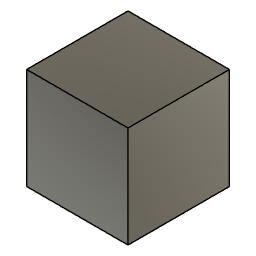
wheel (Autodesk Fusion 360 archive; units mm, degrees)
design "휠 기준점"
Autodesk Fusion 360 part; units mm, degrees
sketch "스케치1" plane through (0, 0, 0) normal (0, 0, 1) x (1, 0, 0)
  line L0 (0, 0) -> (-3, 0)
  line L1 (-3, 0) -> (-3, 3)
  line L2 (-3, 3) -> (0, 3)
  line L3 (0, 3) -> (0, 0)
  dimension "d1" = 3
  dimension "d2" = 3
  constraint horizontal L0
  constraint vertical L1
  constraint horizontal L2
  constraint vertical L3
  constraint coincident L0.start L3.end
  measures "d1" distance of L0.start L0.end
  measures "d2" distance of L0.start L2.end
extrude "돌출1" add sketch "스케치1" along normal blind 3

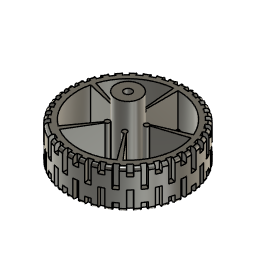
design "휠"
Autodesk Fusion 360 part; units mm, degrees
sketch "스케치1" plane through (0, 0, 0) normal (0, 0, 1) x (1, 0, 0)
  circle A0 centre (0, 0) radius 62.5
  dimension "d1" = 125
  constraint coincident A0.centre origin
  measures "d1" diameter of A0
extrude "돌출1" add sketch "스케치1" along normal blind 40
sketch "스케치2" plane through (0, 0, 40) normal (0, 0, 1) x (-1, 0, 0)
  circle A0 centre (0, 0) radius 62.5
  circle A1 centre (0, 0) radius 13
  dimension "d4" = 26
  constraint coincident A0.centre A1.centre
  measures "d4" diameter of A1
extrude "돌출2" add sketch "스케치2" along normal blind 25.5 contours A1
sketch "스케치3" plane through (0, 0, 65.5) normal (0, 0, 1) x (-1, 0, 0)
  circle A0 centre (0, 0) radius 13
  circle A1 centre (0, 0) radius 4
  dimension "d7" = 8
  constraint coincident A0.centre A1.centre
  measures "d7" diameter of A1
extrude "돌출3" cut sketch "스케치3" against normal blind 20.5 contours A1
sketch "스케치6" plane through (0, 0, 0) normal (0, 0, 1) x (1, 0, 0)
  circle A0 centre (0, 0) radius 18
  circle A1 centre (0, 0) radius 21
  circle A2 centre (0, 0) radius 55
  circle A3 centre (0, 0) radius 52.5
  line L0 (0, 0) -> (0, 52.5)
  line L1 (0, 0) -> (49.9305, 16.2234)
  line L2 (0, 0) -> (30.8587, -42.4734)
  line L3 (0, 0) -> (-30.8587, -42.4734)
  line L4 (0, 0) -> (-49.9305, 16.2234)
  line L5 (0, 21) -> (10, 21)
  line L6 (10, 21) -> (0, 52.5)
  line L7 (10, 21) -> (37.4155, 36.8284)
  line L8 (10, 21) -> (40.9959, 21) construction
  line L9 (19.9722, 6.4894) -> (23.0624, -3.0212)
  line L10 (23.0624, -3.0212) -> (49.9305, 16.2234)
  line L11 (23.0624, -3.0212) -> (46.5879, -24.2037)
  line L12 (12.3435, -16.9894) -> (4.2533, -22.8672)
  line L13 (4.2533, -22.8672) -> (30.8587, -42.4734)
  line L14 (4.2533, -22.8672) -> (-8.6226, -51.7871)
  line L15 (-12.3435, -16.9894) -> (-20.4337, -11.1115)
  line L16 (-20.4337, -11.1115) -> (-30.8587, -42.4734)
  line L17 (-20.4337, -11.1115) -> (-51.917, -7.8025)
  line L18 (-19.9722, 6.4894) -> (-16.882, 15.9999)
  line L19 (-16.882, 15.9999) -> (-49.9305, 16.2234)
  line L20 (-16.882, 15.9999) -> (-23.4638, 46.9649)
  line L21 (-16.882, 15.9999) -> (14.7747, 15.9999) construction
  dimension "d41" = 108
  dimension "d46" = 30
  constraint coincident A0.centre A1.centre
  constraint concentric A0 A2
  constraint coincident A3 L0.end
  constraint vertical L0
  constraint coincident A3 L1.end
  constraint coincident A3 L2.end
  constraint coincident A3 L3.end
  constraint coincident A3 L4.end
  constraint coincident L0 L5.start
  constraint coincident A1 L5.start
  constraint perpendicular L0 L5
  constraint horizontal L8
  constraint coincident A3 L7.end
  constraint coincident A1 L9.start
  constraint coincident L1 L9.start
  constraint tangent A1 L9
  constraint coincident A3 L11.end
  constraint coincident A1 L12.start
  constraint coincident L2 L12.start
  constraint tangent A1 L12
  constraint coincident A3 L14.end
  constraint coincident L3 L15.start
  constraint coincident A1 L15.start
  constraint perpendicular L3 L15
  constraint coincident A3 L17.end
  constraint coincident L4 L18.start
  constraint coincident A1 L18.start
  constraint perpendicular L4 L18
  constraint horizontal L21
  constraint coincident A3 L20.end
  measures "d41" angle of L0 L1
  measures "d46" angle of L7 L8
extrude "돌출6" cut sketch "스케치6" along normal blind 75 contours A3 L10 L11 | A3 L13 L14 | A3 L6 L7 | A3 L16 L17 | A3 L19 L20
extrude "돌출7" add sketch "스케치6" against normal blind 1 contours A0 L1 L2 | A0 L0 L1 | A0 L2 L3 | A0 L0 L4 | A0 L3 L4
fillet "모깎기1" radius 0.5 1 edges at (-16.7819, 6.5091, -1)
sketch "스케치7" plane through (0, 0, 0) normal (0, 0, -1) x (1, 0, 0)
  circle A0 centre (0, 0) radius 18
  line L0 (30.8587, 42.4734) -> (4.2533, 22.8672)
  line L1 (4.2533, 22.8672) -> (-8.6226, 51.7871)
  arc A1 (30.8587, 42.4734) -> (-8.6226, 51.7871) centre (0, 0) ccw
  line L2 (49.9305, -16.2234) -> (23.0624, 3.0212)
  line L3 (23.0624, 3.0212) -> (46.5879, 24.2037)
  arc A2 (49.9305, -16.2234) -> (46.5879, 24.2037) centre (0, 0) ccw
  line L4 (-49.9305, -16.2234) -> (-16.882, -15.9999)
  line L5 (-16.882, -15.9999) -> (-23.4638, -46.9649)
  arc A3 (-49.9305, -16.2234) -> (-23.4638, -46.9649) centre (0, 0) ccw
  line L6 (0, -52.5) -> (10, -21)
  line L7 (10, -21) -> (37.4155, -36.8284)
  arc A4 (0, -52.5) -> (37.4155, -36.8284) centre (0, 0) ccw
  line L8 (-30.8587, 42.4734) -> (-20.4337, 11.1115)
  line L9 (-20.4337, 11.1115) -> (-51.917, 7.8025)
  arc A5 (-30.8587, 42.4734) -> (-51.917, 7.8025) centre (0, 0) ccw
  circle A6 centre (0, 0) radius 62.5
  circle A7 centre (0, 0) radius 57.5
  circle A8 centre (0, 0) radius 62.5
  line L10 (0, 0) -> (-1.368, 1.8829)
  line L11 (0, 0) -> (-30.8587, 42.4734)
  line L12 (-30.8587, 42.4734) -> (-36.7366, 50.5636)
  line L13 (-34.4431, 39.6223) -> (-41.0037, 47.1693)
  line L14 (-37.7653, 36.4696) -> (-44.9587, 43.4161)
  line L15 (-40.8002, 33.0393) -> (-48.5716, 39.3325)
  line L16 (-43.5245, 29.3576) -> (-51.8148, 34.9496)
  line L17 (-45.9175, 25.4525) -> (-54.6637, 30.3006)
  line L18 (-47.9611, 21.3537) -> (-57.0966, 25.421)
  line L19 (-49.6397, 17.0923) -> (-59.0949, 20.348)
  line L20 (-50.9405, 12.7009) -> (-60.6435, 15.1201)
  line L21 (-51.8536, 8.2128) -> (-61.7305, 9.7772)
  line L22 (-52.3721, 3.6622) -> (-62.3478, 4.3598)
  line L23 (-52.492, -0.9163) -> (-62.4905, -1.0908)
  line L24 (-52.2124, -5.4877) -> (-62.1576, -6.533)
  line L25 (-51.5354, -10.0175) -> (-61.3517, -11.9256)
  line L26 (-50.4662, -14.471) -> (-60.0789, -17.2273)
  line L27 (-49.013, -18.8143) -> (-58.3488, -22.398)
  line L28 (-47.1867, -23.0145) -> (-56.1746, -27.3982)
  line L29 (-45.0013, -27.0395) -> (-53.573, -32.1899)
  line L30 (-42.4734, -30.8587) -> (-50.5636, -36.7366)
  line L31 (-39.6223, -34.4431) -> (-47.1693, -41.0037)
  line L32 (-36.4696, -37.7653) -> (-43.4161, -44.9587)
  line L33 (-33.0393, -40.8002) -> (-39.3325, -48.5716)
  line L34 (-29.3576, -43.5245) -> (-34.9496, -51.8148)
  line L35 (-25.4525, -45.9175) -> (-30.3006, -54.6637)
  line L36 (-21.3537, -47.9611) -> (-25.421, -57.0966)
  line L37 (-17.0923, -49.6397) -> (-20.348, -59.0949)
  line L38 (-12.7009, -50.9405) -> (-15.1201, -60.6435)
  line L39 (-8.2128, -51.8536) -> (-9.7772, -61.7305)
  line L40 (-3.6622, -52.3721) -> (-4.3598, -62.3478)
  line L41 (0.9163, -52.492) -> (1.0908, -62.4905)
  line L42 (5.4877, -52.2124) -> (6.533, -62.1576)
  line L43 (10.0175, -51.5354) -> (11.9256, -61.3517)
  line L44 (14.471, -50.4662) -> (17.2273, -60.0789)
  line L45 (18.8143, -49.013) -> (22.398, -58.3488)
  line L46 (23.0145, -47.1867) -> (27.3982, -56.1746)
  line L47 (27.0395, -45.0013) -> (32.1899, -53.573)
  line L48 (30.8587, -42.4734) -> (36.7366, -50.5636)
  line L49 (34.4431, -39.6223) -> (41.0037, -47.1693)
  line L50 (37.7653, -36.4696) -> (44.9587, -43.4161)
  line L51 (40.8002, -33.0393) -> (48.5716, -39.3325)
  line L52 (43.5245, -29.3576) -> (51.8148, -34.9496)
  line L53 (45.9175, -25.4525) -> (54.6637, -30.3006)
  line L54 (47.9611, -21.3537) -> (57.0966, -25.421)
  line L55 (49.6397, -17.0923) -> (59.0949, -20.348)
  line L56 (50.9405, -12.7009) -> (60.6435, -15.1201)
  line L57 (51.8536, -8.2128) -> (61.7305, -9.7772)
  line L58 (52.3721, -3.6622) -> (62.3478, -4.3598)
  line L59 (52.492, 0.9163) -> (62.4905, 1.0908)
  line L60 (52.2124, 5.4877) -> (62.1576, 6.533)
  line L61 (51.5354, 10.0175) -> (61.3517, 11.9256)
  line L62 (50.4662, 14.471) -> (60.0789, 17.2273)
  line L63 (49.013, 18.8143) -> (58.3488, 22.398)
  line L64 (47.1867, 23.0145) -> (56.1746, 27.3982)
  line L65 (45.0013, 27.0395) -> (53.573, 32.1899)
  line L66 (42.4734, 30.8587) -> (50.5636, 36.7366)
  line L67 (39.6223, 34.4431) -> (47.1693, 41.0037)
  line L68 (36.4696, 37.7653) -> (43.4161, 44.9587)
  line L69 (33.0393, 40.8002) -> (39.3325, 48.5716)
  line L70 (29.3576, 43.5245) -> (34.9496, 51.8148)
  line L71 (25.4525, 45.9175) -> (30.3006, 54.6637)
  line L72 (21.3537, 47.9611) -> (25.421, 57.0966)
  line L73 (17.0923, 49.6397) -> (20.348, 59.0949)
  line L74 (12.7009, 50.9405) -> (15.1201, 60.6435)
  line L75 (8.2128, 51.8536) -> (9.7772, 61.7305)
  line L76 (3.6622, 52.3721) -> (4.3598, 62.3478)
  line L77 (-0.9163, 52.492) -> (-1.0908, 62.4905)
  line L78 (-5.4877, 52.2124) -> (-6.533, 62.1576)
  line L79 (-10.0175, 51.5354) -> (-11.9256, 61.3517)
  line L80 (-14.471, 50.4662) -> (-17.2273, 60.0789)
  line L81 (-18.8143, 49.013) -> (-22.398, 58.3488)
  line L82 (-23.0145, 47.1867) -> (-27.3982, 56.1746)
  line L83 (-27.0395, 45.0013) -> (-32.1899, 53.573)
  dimension "d61" = 115
  dimension "d62" = 125
  dimension "d64" = 360
  constraint coincident A0.centre A1.centre
  constraint concentric A7 A8
  constraint coincident L8.start A5.start
  constraint coincident A8 L12.end
  constraint parallel L11 L12
  measures "d61" diameter of A7
  measures "d62" diameter of A8
fillet "모깎기2" radius 3 1 edges at (-58.2705, -22.601, 0)
extrude "돌출8" cut sketch "스케치7" against normal blind 20 contours A6 A7 A8 L71 L72 | A6 A7 A8 L67 L68 | A6 A7 A8 L79 L80 | A6 A7 A8 L75 L76 | A6 A7 A8 L63 L64 | A6 A7 A8 L12 L83 | A6 A7 A8 L59 L60 | A6 A7 A8 L15 L16 | A6 A7 A8 L55 L56 | A6 A7 A8 L19 L20 | A6 A7 A8 L23 L24 | A6 A7 A8 L51 L52 | A6 A7 A8 L27 L28 | A6 A7 A8 L47 L48 | A6 A7 A8 L31 L32 | A6 A7 A8 L43 L44 | A6 A7 A8 L35 L36 | A6 A7 A8 L39 L40
extrude "돌출9" cut sketch "스케치7" against normal blind 8 contours A6 A7 A8 L69 L70 | A6 A7 A8 L77 L78 | A6 A7 A8 L73 L74 | A6 A7 A8 L65 L66 | A6 A7 A8 L81 L82 | A6 A7 A8 L61 L62 | A6 A7 A8 L13 L14 | A6 A7 A8 L17 L18 | A6 A7 A8 L21 L22 | A6 A7 A8 L57 L58 | A6 A7 A8 L53 L54 | A6 A7 A8 L25 L26 | A6 A7 A8 L49 L50 | A6 A7 A8 L29 L30 | A6 A7 A8 L45 L46 | A6 A7 A8 L33 L34 | A6 A7 A8 L41 L42 | A6 A7 A8 L37 L38
sketch "스케치8" plane through (0, 0, 40) normal (0, 0, 1) x (-1, 0, 0)
  line L0 (-4.2533, 22.8672) -> (-30.8587, 42.4734)
  arc A0 (8.6226, 51.7871) -> (-30.8587, 42.4734) centre (0, 0) ccw
  line L1 (8.6226, 51.7871) -> (-4.2533, 22.8672)
  line L2 (-23.0624, 3.0212) -> (-49.9305, -16.2234)
  arc A1 (-46.5879, 24.2037) -> (-49.9305, -16.2234) centre (0, 0) ccw
  line L3 (-46.5879, 24.2037) -> (-23.0624, 3.0212)
  line L4 (16.882, -15.9999) -> (49.9305, -16.2234)
  arc A2 (23.4638, -46.9649) -> (49.9305, -16.2234) centre (0, 0) ccw
  line L5 (23.4638, -46.9649) -> (16.882, -15.9999)
  line L6 (-10, -21) -> (0, -52.5)
  arc A3 (-37.4155, -36.8284) -> (0, -52.5) centre (0, 0) ccw
  line L7 (-37.4155, -36.8284) -> (-10, -21)
  line L8 (20.4337, 11.1115) -> (30.8587, 42.4734)
  arc A4 (51.917, 7.8025) -> (30.8587, 42.4734) centre (0, 0) ccw
  line L9 (51.917, 7.8025) -> (20.4337, 11.1115)
  circle A5 centre (0, 0) radius 13
  circle A6 centre (0, 0) radius 62.5
  circle A7 centre (0, 0) radius 62.5
  circle A8 centre (0, 0) radius 57.5
  line L10 (0, 0) -> (0, -1.8263)
  line L11 (0, -1.8263) -> (23.4638, -46.9649)
  line L12 (0, 0) -> (30.8587, 42.4734)
  line L13 (30.8587, 42.4734) -> (36.7366, 50.5636)
  line L14 (27.0395, 45.0013) -> (32.1899, 53.573)
  line L15 (23.0145, 47.1867) -> (27.3982, 56.1746)
  line L16 (18.8143, 49.013) -> (22.398, 58.3488)
  line L17 (14.471, 50.4662) -> (17.2273, 60.0789)
  line L18 (10.0175, 51.5354) -> (11.9256, 61.3517)
  line L19 (5.4877, 52.2124) -> (6.533, 62.1576)
  line L20 (0.9163, 52.492) -> (1.0908, 62.4905)
  line L21 (-3.6622, 52.3721) -> (-4.3598, 62.3478)
  line L22 (-8.2128, 51.8536) -> (-9.7772, 61.7305)
  line L23 (-12.7009, 50.9405) -> (-15.1201, 60.6435)
  line L24 (-17.0923, 49.6397) -> (-20.348, 59.0949)
  line L25 (-21.3537, 47.9611) -> (-25.421, 57.0966)
  line L26 (-25.4525, 45.9175) -> (-30.3006, 54.6637)
  line L27 (-29.3576, 43.5245) -> (-34.9496, 51.8148)
  line L28 (-33.0393, 40.8002) -> (-39.3325, 48.5716)
  line L29 (-36.4696, 37.7653) -> (-43.4161, 44.9587)
  line L30 (-39.6223, 34.4431) -> (-47.1693, 41.0037)
  line L31 (-42.4734, 30.8587) -> (-50.5636, 36.7366)
  line L32 (-45.0013, 27.0395) -> (-53.573, 32.1899)
  line L33 (-47.1867, 23.0145) -> (-56.1746, 27.3982)
  line L34 (-49.013, 18.8143) -> (-58.3488, 22.398)
  line L35 (-50.4662, 14.471) -> (-60.0789, 17.2273)
  line L36 (-51.5354, 10.0175) -> (-61.3517, 11.9256)
  line L37 (-52.2124, 5.4877) -> (-62.1576, 6.533)
  line L38 (-52.492, 0.9163) -> (-62.4905, 1.0908)
  line L39 (-52.3721, -3.6622) -> (-62.3478, -4.3598)
  line L40 (-51.8536, -8.2128) -> (-61.7305, -9.7772)
  line L41 (-50.9405, -12.7009) -> (-60.6435, -15.1201)
  line L42 (-49.6397, -17.0923) -> (-59.0949, -20.348)
  line L43 (-47.9611, -21.3537) -> (-57.0966, -25.421)
  line L44 (-45.9175, -25.4525) -> (-54.6637, -30.3006)
  line L45 (-43.5245, -29.3576) -> (-51.8148, -34.9496)
  line L46 (-40.8002, -33.0393) -> (-48.5716, -39.3325)
  line L47 (-37.7653, -36.4696) -> (-44.9587, -43.4161)
  line L48 (-34.4431, -39.6223) -> (-41.0037, -47.1693)
  line L49 (-30.8587, -42.4734) -> (-36.7366, -50.5636)
  line L50 (-27.0395, -45.0013) -> (-32.1899, -53.573)
  line L51 (-23.0145, -47.1867) -> (-27.3982, -56.1746)
  line L52 (-18.8143, -49.013) -> (-22.398, -58.3488)
  line L53 (-14.471, -50.4662) -> (-17.2273, -60.0789)
  line L54 (-10.0175, -51.5354) -> (-11.9256, -61.3517)
  line L55 (-5.4877, -52.2124) -> (-6.533, -62.1576)
  line L56 (-0.9163, -52.492) -> (-1.0908, -62.4905)
  line L57 (3.6622, -52.3721) -> (4.3598, -62.3478)
  line L58 (8.2128, -51.8536) -> (9.7772, -61.7305)
  line L59 (12.7009, -50.9405) -> (15.1201, -60.6435)
  line L60 (17.0923, -49.6397) -> (20.348, -59.0949)
  line L61 (21.3537, -47.9611) -> (25.421, -57.0966)
  line L62 (25.4525, -45.9175) -> (30.3006, -54.6637)
  line L63 (29.3576, -43.5245) -> (34.9496, -51.8148)
  line L64 (33.0393, -40.8002) -> (39.3325, -48.5716)
  line L65 (36.4696, -37.7653) -> (43.4161, -44.9587)
  line L66 (39.6223, -34.4431) -> (47.1693, -41.0037)
  line L67 (42.4734, -30.8587) -> (50.5636, -36.7366)
  line L68 (45.0013, -27.0395) -> (53.573, -32.1899)
  line L69 (47.1867, -23.0145) -> (56.1746, -27.3982)
  line L70 (49.013, -18.8143) -> (58.3488, -22.398)
  line L71 (50.4662, -14.471) -> (60.0789, -17.2273)
  line L72 (51.5354, -10.0175) -> (61.3517, -11.9256)
  line L73 (52.2124, -5.4877) -> (62.1576, -6.533)
  line L74 (52.492, -0.9163) -> (62.4905, -1.0908)
  line L75 (52.3721, 3.6622) -> (62.3478, 4.3598)
  line L76 (51.8536, 8.2128) -> (61.7305, 9.7772)
  line L77 (50.9405, 12.7009) -> (60.6435, 15.1201)
  line L78 (49.6397, 17.0923) -> (59.0949, 20.348)
  line L79 (47.9611, 21.3537) -> (57.0966, 25.421)
  line L80 (45.9175, 25.4525) -> (54.6637, 30.3006)
  line L81 (43.5245, 29.3576) -> (51.8148, 34.9496)
  line L82 (40.8002, 33.0393) -> (48.5716, 39.3325)
  line L83 (37.7653, 36.4696) -> (44.9587, 43.4161)
  line L84 (34.4431, 39.6223) -> (41.0037, 47.1693)
  dimension "d74" = 360
  constraint coincident A0.centre A1.centre
  constraint concentric A7 A8
  constraint vertical L10
  constraint coincident A2.start L5.start
  constraint coincident L8.end A4.end
  constraint coincident A7 L13.end
  constraint parallel L12 L13
fillet "모깎기3" radius 3 1 edges at (-58.2705, -22.601, 40)
extrude "돌출10" cut sketch "스케치8" against normal blind 20 contours A6 A7 A8 L27 L28 | A6 A7 A8 L19 L20 | A6 A7 A8 L23 L24 | A6 A7 A8 L15 L16 | A6 A7 A8 L31 L32 | A6 A7 A8 L83 L84 | A6 A7 A8 L35 L36 | A6 A7 A8 L79 L80 | A6 A7 A8 L75 L76 | A6 A7 A8 L39 L40 | A6 A7 A8 L63 L64 | A6 A7 A8 L43 L44 | A6 A7 A8 L59 L60 | A6 A7 A8 L71 L72 | A6 A7 A8 L67 L68 | A6 A7 A8 L47 L48 | A6 A7 A8 L55 L56 | A6 A7 A8 L51 L52
extrude "돌출11" cut sketch "스케치8" against normal blind 8 contours A6 A7 A8 L25 L26 | A6 A7 A8 L17 L18 | A6 A7 A8 L29 L30 | A6 A7 A8 L21 L22 | A6 A7 A8 L33 L34 | A6 A7 A8 L81 L82 | A6 A7 A8 L37 L38 | A6 A7 A8 L41 L42 | A6 A7 A8 L77 L78 | A6 A7 A8 L61 L62 | A6 A7 A8 L73 L74 | A6 A7 A8 L69 L70 | A6 A7 A8 L65 L66 | A6 A7 A8 L45 L46 | A6 A7 A8 L57 L58 | A6 A7 A8 L49 L50 | A6 A7 A8 L53 L54
sketch "스케치9" plane through (0, 0, 40) normal (0, 0, 1) x (-1, 0, 0)
  line L0 (53.6809, -20.6062) -> (55.548, -21.3229)
  arc A0 (55.548, -21.3229) -> (57.1951, -16.4004) centre (0, 0) ccw
  line L1 (57.1951, -16.4004) -> (55.2725, -15.8491)
  arc A1 (55.2725, -15.8491) -> (56.4436, -10.9715) centre (0, 0) ccw
  line L2 (56.4436, -10.9715) -> (58.4068, -11.3531)
  arc A2 (58.4068, -11.3531) -> (59.1741, -6.2194) centre (0, 0) ccw
  line L3 (59.1741, -6.2194) -> (57.185, -6.0104)
  arc A3 (57.185, -6.0104) -> (57.4912, -1.0035) centre (0, 0) ccw
  line L4 (57.4912, -1.0035) -> (59.4909, -1.0384)
  arc A4 (59.4909, -1.0384) -> (59.3551, 4.1505) centre (0, 0) ccw
  line L5 (59.3551, 4.1505) -> (57.3599, 4.011)
  arc A5 (57.3599, 4.011) -> (56.7921, 8.995) centre (0, 0) ccw
  line L6 (56.7921, 8.995) -> (58.7675, 9.3079)
  arc A6 (58.7675, 9.3079) -> (57.7326, 14.3944) centre (0, 0) ccw
  line L7 (57.7326, 14.3944) -> (55.792, 13.9105)
  arc A7 (55.792, 13.9105) -> (54.3673, 18.7202) centre (0, 0) ccw
  line L8 (54.3673, 18.7202) -> (56.2584, 19.3713)
  arc A8 (56.2584, 19.3713) -> (54.356, 24.2008) centre (0, 0) ccw
  line L9 (54.356, 24.2008) -> (52.5289, 23.3874)
  arc A9 (52.5289, 23.3874) -> (50.2906, 27.8766) centre (0, 0) ccw
  line L10 (50.2906, 27.8766) -> (52.0399, 28.8462)
  arc A10 (52.0399, 28.8462) -> (49.3277, 33.272) centre (0, 0) ccw
  line L11 (49.3277, 33.272) -> (47.6697, 32.1536)
  arc A11 (47.6697, 32.1536) -> (44.6859, 36.1859) centre (0, 0) ccw
  line L12 (44.6859, 36.1859) -> (46.2402, 37.4446)
  arc A12 (46.2402, 37.4446) -> (42.8007, 41.3322) centre (0, 0) ccw
  line L13 (42.8007, 41.3322) -> (41.362, 39.9429)
  arc A13 (41.362, 39.9429) -> (37.7234, 43.3958) centre (0, 0) ccw
  line L14 (37.7234, 43.3958) -> (39.0355, 44.9052)
  arc A14 (39.0355, 44.9052) -> (26.0831, 53.4782) centre (0, 0) ccw
  line L15 (26.0831, 53.4782) -> (25.2063, 51.6807)
  arc A15 (25.2063, 51.6807) -> (20.6062, 53.6809) centre (0, 0) ccw
  line L16 (20.6062, 53.6809) -> (21.3229, 55.548)
  arc A16 (21.3229, 55.548) -> (16.4004, 57.1951) centre (0, 0) ccw
  line L17 (16.4004, 57.1951) -> (15.8491, 55.2725)
  arc A17 (15.8491, 55.2725) -> (10.9715, 56.4436) centre (0, 0) ccw
  line L18 (10.9715, 56.4436) -> (11.3531, 58.4068)
  arc A18 (11.3531, 58.4068) -> (6.2194, 59.1741) centre (0, 0) ccw
  line L19 (6.2194, 59.1741) -> (6.0104, 57.185)
  arc A19 (6.0104, 57.185) -> (1.0035, 57.4912) centre (0, 0) ccw
  line L20 (1.0035, 57.4912) -> (1.0384, 59.4909)
  arc A20 (1.0384, 59.4909) -> (-4.1505, 59.3551) centre (0, 0) ccw
  line L21 (-4.1505, 59.3551) -> (-4.011, 57.3599)
  arc A21 (-4.011, 57.3599) -> (-8.995, 56.7921) centre (0, 0) ccw
  line L22 (-8.995, 56.7921) -> (-9.3079, 58.7675)
  arc A22 (-9.3079, 58.7675) -> (-14.3944, 57.7326) centre (0, 0) ccw
  line L23 (-14.3944, 57.7326) -> (-13.9105, 55.792)
  arc A23 (-13.9105, 55.792) -> (-18.7202, 54.3673) centre (0, 0) ccw
  line L24 (-18.7202, 54.3673) -> (-19.3713, 56.2584)
  arc A24 (-19.3713, 56.2584) -> (-24.2008, 54.356) centre (0, 0) ccw
  line L25 (-24.2008, 54.356) -> (-23.3874, 52.5289)
  arc A25 (-23.3874, 52.5289) -> (-27.8766, 50.2906) centre (0, 0) ccw
  line L26 (-27.8766, 50.2906) -> (-28.8462, 52.0399)
  arc A26 (-28.8462, 52.0399) -> (-33.272, 49.3277) centre (0, 0) ccw
  line L27 (-33.272, 49.3277) -> (-32.1536, 47.6697)
  arc A27 (-32.1536, 47.6697) -> (-36.1859, 44.6859) centre (0, 0) ccw
  line L28 (-36.1859, 44.6859) -> (-37.4446, 46.2402)
  arc A28 (-37.4446, 46.2402) -> (-41.3322, 42.8007) centre (0, 0) ccw
  line L29 (-41.3322, 42.8007) -> (-39.9429, 41.362)
  arc A29 (-39.9429, 41.362) -> (-43.3958, 37.7234) centre (0, 0) ccw
  line L30 (-43.3958, 37.7234) -> (-44.9052, 39.0355)
  arc A30 (-44.9052, 39.0355) -> (-48.1365, 34.9732) centre (0, 0) ccw
  line L31 (-48.1365, 34.9732) -> (-46.5185, 33.7977)
  arc A31 (-46.5185, 33.7977) -> (-49.2871, 29.6147) centre (0, 0) ccw
  line L32 (-49.2871, 29.6147) -> (-51.0015, 30.6448)
  arc A32 (-51.0015, 30.6448) -> (-53.4782, 26.0831) centre (0, 0) ccw
  line L33 (-53.4782, 26.0831) -> (-51.6807, 25.2063)
  arc A33 (-51.6807, 25.2063) -> (-53.6809, 20.6062) centre (0, 0) ccw
  line L34 (-53.6809, 20.6062) -> (-55.548, 21.3229)
  arc A34 (-55.548, 21.3229) -> (-57.1951, 16.4004) centre (0, 0) ccw
  line L35 (-57.1951, 16.4004) -> (-55.2725, 15.8491)
  arc A35 (-55.2725, 15.8491) -> (-56.4436, 10.9715) centre (0, 0) ccw
  line L36 (-56.4436, 10.9715) -> (-58.4068, 11.3531)
  arc A36 (-58.4068, 11.3531) -> (-59.1741, 6.2194) centre (0, 0) ccw
  line L37 (-59.1741, 6.2194) -> (-57.185, 6.0104)
  arc A37 (-57.185, 6.0104) -> (-57.4912, 1.0035) centre (0, 0) ccw
  line L38 (-57.4912, 1.0035) -> (-59.4909, 1.0384)
  arc A38 (-59.4909, 1.0384) -> (-59.3551, -4.1505) centre (0, 0) ccw
  line L39 (-59.3551, -4.1505) -> (-57.3599, -4.011)
  arc A39 (-57.3599, -4.011) -> (-56.7921, -8.995) centre (0, 0) ccw
  line L40 (-56.7921, -8.995) -> (-58.7675, -9.3079)
  arc A40 (-58.7675, -9.3079) -> (-57.7326, -14.3944) centre (0, 0) ccw
  line L41 (-57.7326, -14.3944) -> (-55.792, -13.9105)
  arc A41 (-55.792, -13.9105) -> (-54.3673, -18.7202) centre (0, 0) ccw
  line L42 (-54.3673, -18.7202) -> (-56.2584, -19.3713)
  arc A42 (-56.2584, -19.3713) -> (-54.356, -24.2008) centre (0, 0) ccw
  line L43 (-54.356, -24.2008) -> (-52.5289, -23.3874)
  arc A43 (-52.5289, -23.3874) -> (-50.2906, -27.8766) centre (0, 0) ccw
  line L44 (-50.2906, -27.8766) -> (-52.0399, -28.8462)
  arc A44 (-52.0399, -28.8462) -> (-49.3277, -33.272) centre (0, 0) ccw
  line L45 (-49.3277, -33.272) -> (-47.6697, -32.1536)
  arc A45 (-47.6697, -32.1536) -> (-44.6859, -36.1859) centre (0, 0) ccw
  line L46 (-44.6859, -36.1859) -> (-46.2402, -37.4446)
  arc A46 (-46.2402, -37.4446) -> (-42.8007, -41.3322) centre (0, 0) ccw
  line L47 (-42.8007, -41.3322) -> (-41.362, -39.9429)
  arc A47 (-41.362, -39.9429) -> (-37.7234, -43.3958) centre (0, 0) ccw
  line L48 (-37.7234, -43.3958) -> (-39.0355, -44.9052)
  arc A48 (-39.0355, -44.9052) -> (-34.9732, -48.1365) centre (0, 0) ccw
  line L49 (-34.9732, -48.1365) -> (-33.7977, -46.5185)
  arc A49 (-33.7977, -46.5185) -> (-29.6147, -49.2871) centre (0, 0) ccw
  line L50 (-29.6147, -49.2871) -> (-30.6448, -51.0015)
  arc A50 (-30.6448, -51.0015) -> (-26.0831, -53.4782) centre (0, 0) ccw
  line L51 (-26.0831, -53.4782) -> (-25.2063, -51.6807)
  arc A51 (-25.2063, -51.6807) -> (-20.6062, -53.6809) centre (0, 0) ccw
  line L52 (-20.6062, -53.6809) -> (-21.3229, -55.548)
  arc A52 (-21.3229, -55.548) -> (-16.4004, -57.1951) centre (0, 0) ccw
  line L53 (-16.4004, -57.1951) -> (-15.8491, -55.2725)
  arc A53 (-15.8491, -55.2725) -> (-10.9715, -56.4436) centre (0, 0) ccw
  line L54 (-10.9715, -56.4436) -> (-11.3531, -58.4068)
  arc A54 (-11.3531, -58.4068) -> (-6.2194, -59.1741) centre (0, 0) ccw
  line L55 (-6.2194, -59.1741) -> (-6.0104, -57.185)
  arc A55 (-6.0104, -57.185) -> (-1.0035, -57.4912) centre (0, 0) ccw
  line L56 (-1.0035, -57.4912) -> (-1.0384, -59.4909)
  arc A56 (-1.0384, -59.4909) -> (4.1505, -59.3551) centre (0, 0) ccw
  line L57 (4.1505, -59.3551) -> (4.011, -57.3599)
  arc A57 (4.011, -57.3599) -> (8.995, -56.7921) centre (0, 0) ccw
  line L58 (8.995, -56.7921) -> (9.3079, -58.7675)
  arc A58 (9.3079, -58.7675) -> (14.3944, -57.7326) centre (0, 0) ccw
  line L59 (14.3944, -57.7326) -> (13.9105, -55.792)
  arc A59 (13.9105, -55.792) -> (18.7202, -54.3673) centre (0, 0) ccw
  line L60 (18.7202, -54.3673) -> (19.3713, -56.2584)
  arc A60 (19.3713, -56.2584) -> (24.2008, -54.356) centre (0, 0) ccw
  line L61 (24.2008, -54.356) -> (23.3874, -52.5289)
  arc A61 (23.3874, -52.5289) -> (27.8766, -50.2906) centre (0, 0) ccw
  line L62 (27.8766, -50.2906) -> (28.8462, -52.0399)
  arc A62 (28.8462, -52.0399) -> (33.272, -49.3277) centre (0, 0) ccw
  line L63 (33.272, -49.3277) -> (32.1536, -47.6697)
  arc A63 (32.1536, -47.6697) -> (36.1859, -44.6859) centre (0, 0) ccw
  line L64 (36.1859, -44.6859) -> (37.4446, -46.2402)
  arc A64 (37.4446, -46.2402) -> (41.3322, -42.8007) centre (0, 0) ccw
  line L65 (41.3322, -42.8007) -> (39.9429, -41.362)
  arc A65 (39.9429, -41.362) -> (43.3958, -37.7234) centre (0, 0) ccw
  line L66 (43.3958, -37.7234) -> (44.9052, -39.0355)
  arc A66 (44.9052, -39.0355) -> (48.1365, -34.9732) centre (0, 0) ccw
  line L67 (48.1365, -34.9732) -> (46.5185, -33.7977)
  arc A67 (46.5185, -33.7977) -> (49.2871, -29.6147) centre (0, 0) ccw
  line L68 (49.2871, -29.6147) -> (51.0015, -30.6448)
  arc A68 (51.0015, -30.6448) -> (53.4782, -26.0831) centre (0, 0) ccw
  line L69 (53.4782, -26.0831) -> (51.6807, -25.2063)
  arc A69 (51.6807, -25.2063) -> (53.6809, -20.6062) centre (0, 0) ccw
  circle A70 centre (0, 0) radius 13
  line L70 (20.4337, 11.1115) -> (30.8587, 42.4734)
  arc A71 (51.917, 7.8025) -> (30.8587, 42.4734) centre (0, 0) ccw
  line L71 (51.917, 7.8025) -> (20.4337, 11.1115)
  line L72 (-10, -21) -> (0, -52.5)
  arc A72 (-37.4155, -36.8284) -> (0, -52.5) centre (0, 0) ccw
  line L73 (-37.4155, -36.8284) -> (-10, -21)
  line L74 (16.882, -15.9999) -> (49.9305, -16.2234)
  arc A73 (23.4638, -46.9649) -> (49.9305, -16.2234) centre (0, 0) ccw
  line L75 (23.4638, -46.9649) -> (16.882, -15.9999)
  line L76 (-23.0624, 3.0212) -> (-49.9305, -16.2234)
  arc A74 (-46.5879, 24.2037) -> (-49.9305, -16.2234) centre (0, 0) ccw
  line L77 (-46.5879, 24.2037) -> (-23.0624, 3.0212)
  line L78 (-4.2533, 22.8672) -> (-30.8587, 42.4734)
  arc A75 (8.6226, 51.7871) -> (-30.8587, 42.4734) centre (0, 0) ccw
  line L79 (8.6226, 51.7871) -> (-4.2533, 22.8672)
  circle A76 centre (0, 0) radius 52.5
  line L80 (0, 0) -> (0, 5)
  line L81 (-30.8587, 42.4734) -> (0, 0)
  line L82 (-49.9305, -16.2234) -> (0, 0)
  line L83 (0, 0) -> (0, -52.5)
  line L84 (0, 0) -> (49.9305, -16.2234)
  line L85 (0, 0) -> (30.8587, 42.4734)
  line L86 (-7.6412, 10.5172) -> (-9.1107, 12.5398)
  circle A77 centre (-9.1107, 12.5398) radius 2.5
  circle A78 centre (-14.7414, -4.7898) radius 2.5
  circle A79 centre (0, -15.5) radius 2.5
  circle A80 centre (14.7414, -4.7898) radius 2.5
  circle A81 centre (9.1107, 12.5398) radius 2.5
  line L87 (0, 0) -> (-34.4431, 39.6223)
  line L88 (0, 0) -> (52.5, 0) construction
  line L89 (0, 0) -> (-48.3265, -20.5134)
  line L90 (0, 0) -> (4.5757, -52.3002)
  line L91 (0, 0) -> (51.1544, -11.8099)
  line L92 (0, 0) -> (27.0395, 45.0013)
  dimension "d81" = 2.5
  dimension "d83" = 360
  dimension "d86" = 360
  constraint concentric A0 A76
  constraint coincident A0.centre A1.centre
  constraint vertical L80
  constraint coincident L78.end A75.end
  constraint coincident L76.end A74.end
  constraint coincident L72.end A72.end
  constraint coincident L74.end A73.end
  constraint coincident L70.end A71.end
  constraint coincident A70 L86.start
  constraint coincident L81 L86.start
  constraint parallel L81 L86
  constraint coincident L86.end A77.centre
  constraint coincident L86.start A77
  constraint horizontal L88
  constraint coincident A76 L87.end
  measures "d81" distance of L86.start L86.end
extrude "돌출12" cut sketch "스케치9" against normal blind 35 contours A70 L70 L71 A76 L85 A80 A81 L91 | A70 L78 L79 A76 L81 A77 A81 L92 | A70 L74 L75 A76 L84 A79 A80 L90 | A70 L76 L77 A76 L82 A77 A78 L87 | A70 L72 L73 A76 L83 A78 A79 L89
fillet "모깎기4" radius 2 5 edges at (-20.4337, -11.1115, 2.5) (4.2533, -22.8672, 2.5) (23.0624, -3.0212, 2.5) (10, 21, 2.5) (-16.882, 15.9999, 2.5)
fillet "모깎기5" radius 2 5 edges at (-51.917, -7.8025, 2.5) (-8.6226, -51.7871, 2.5) (46.5879, -24.2037, 2.5) (37.4155, 36.8284, 2.5) (-23.4638, 46.9649, 2.5)
fillet "모깎기6" radius 2 5 edges at (30.8587, -42.4734, 2.5) (49.9305, 16.2234, 2.5) (0, 52.5, 2.5) (-49.9305, 16.2234, 2.5) (-30.8587, -42.4734, 2.5)
